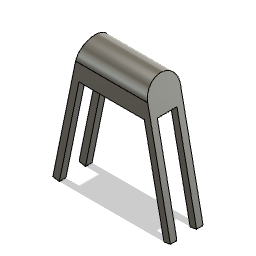
test_7 v2 (Autodesk Fusion 360 design; units mm, degrees)
Autodesk Fusion 360 part; units mm, degrees
sketch "Sketch1" plane through (0, 0, 0) normal (0, 0, 1) x (1, 0, 0)
  line L0 (0, 0) -> (200, 0)
  line L1 (200, 0) -> (200, 100)
  line L2 (200, 100) -> (0, 100)
  line L3 (0, 100) -> (0, 0)
  line L4 (200, 0) -> (219.5959, 4)
  line L5 (200, 100) -> (219.5959, 4)
  line L6 (0, 0) -> (-19.5959, 4)
  line L7 (0, 100) -> (-19.5959, 4)
  dimension "d1" = 200
  dimension "d2" = 100
  dimension "d3" = 20
  dimension "d4" = 20
  constraint horizontal L0
  constraint vertical L1
  constraint horizontal L2
  constraint vertical L3
  constraint coincident L0.start L3.end
  constraint perpendicular L4 L5
  constraint perpendicular L6 L7
  measures "d1" distance of L0.start L0.end
  measures "d2" distance of L0.start L2.end
  measures "d3" distance of L0.end L4.end
  measures "d4" distance of L0.start L6.end
extrude "Extrude1" add sketch "Sketch1" along normal blind 100
sketch "Sketch2" plane through (0, 0, 0) normal (-0.2, -0.979796, 0) x (0, 0, 1)
  line L0 (0, 20) -> (0, 0)
  line L1 (0, 0) -> (100, 0)
  line L2 (100, 0) -> (100, 20)
  line L3 (100, 20) -> (0, 20)
  line L4 (0, 0) -> (20, 0)
  line L5 (20, 0) -> (20, 20)
  line L6 (20, 20) -> (0, 20)
  line L7 (0, 20) -> (0, 0)
  line L8 (100, 0) -> (80, 0)
  line L9 (80, 0) -> (80, 20)
  line L10 (80, 20) -> (100, 20)
  line L11 (100, 20) -> (100, 0)
  dimension "d7" = 20
  dimension "d8" = 20
  dimension "d9" = 20
  dimension "d10" = 20
  constraint horizontal L4
  constraint vertical L5
  constraint horizontal L6
  constraint vertical L7
  constraint coincident L0.end L1.start
  constraint horizontal L8
  constraint vertical L9
  constraint horizontal L10
  constraint vertical L11
  constraint coincident L1.end L2.start
  measures "d7" distance of L0.end L4.end
  measures "d8" distance of L0.end L0.start
  measures "d9" distance of L1.end L8.end
  measures "d10" distance of L1.end L2.end
extrude "Extrude2" add sketch "Sketch2" along normal blind 300 contours L0 L1 L3 L4 L5 L6 L7 | L1 L2 L3 L8 L9 L10 L11
sketch "Sketch3" plane through (8, -39.1918, 0) normal (0.2, -0.979796, 0) x (0, 0, -1)
  line L0 (0, 195.9592) -> (0, 215.9592)
  line L1 (0, 215.9592) -> (-100, 215.9592)
  line L2 (-100, 215.9592) -> (-100, 195.9592)
  line L3 (-100, 195.9592) -> (0, 195.9592)
  line L4 (-100, 195.9592) -> (-80, 195.9592)
  line L5 (-80, 195.9592) -> (-80, 215.9592)
  line L6 (-80, 215.9592) -> (-100, 215.9592)
  line L7 (-100, 215.9592) -> (-100, 195.9592)
  line L8 (0, 195.9592) -> (-20, 195.9592)
  line L9 (-20, 195.9592) -> (-20, 215.9592)
  line L10 (-20, 215.9592) -> (0, 215.9592)
  line L11 (0, 215.9592) -> (0, 195.9592)
  dimension "d13" = 20
  dimension "d14" = 20
  dimension "d15" = 20
  dimension "d16" = 20
  constraint horizontal L4
  constraint vertical L5
  constraint horizontal L6
  constraint vertical L7
  constraint coincident L2.end L3.start
  constraint horizontal L8
  constraint vertical L9
  constraint horizontal L10
  constraint vertical L11
  constraint coincident L0.start L3.end
  measures "d13" distance of L2.end L4.end
  measures "d14" distance of L2.end L1.end
  measures "d15" distance of L0.start L8.end
  measures "d16" distance of L0.start L0.end
extrude "Extrude3" add sketch "Sketch3" along normal blind 300 contours L0 L1 L3 L8 L9 L10 L11 | L1 L2 L3 L4 L5 L6 L7
move_body "Move1" bodies 1 to x (1, 0, 0) y (0, 1, 0) z (0, 0, 1) at (0, 300, 0)
sketch "Sketch4" plane through (0, 0, 0) normal (0, 1, 0) x (1, 0, 0)
fillet "Fillet1" radius 50 2 edges at (100, 400, 0) (100, 400, 100)
